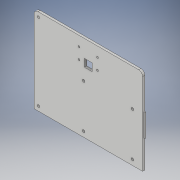
# Autodesk Inventor part: justlid
Saved by Autodesk Inventor 2019 (Build 230136000, 136)
## iProperties
Created: 2019-03-28
Part Number: justlid
Material: Generic
Document SubType Name: Modeling
Designer: eepc07adm
Density: 1 g/cm^3
Appearance: Default
Author: eepc07adm
Autodesk Inventor part; units mm, degrees
ref_plane "YZ Plane" through (0, 0, 0) normal (1, 0, 0) x (0, 1, 0)
ref_plane "XZ Plane" through (0, 0, 0) normal (0, 1, 0) x (-1, 0, 0)
ref_plane "XY Plane" through (0, 0, 0) normal (0, 0, 1) x (1, 0, 0)
sketch "Sketch1" plane through (0, 0, 0) normal (0, 0, 1) x (1, 0, 0)
  line L0 (0, 126.4897) -> (121.92, 126.4897)
  line L1 (121.92, 126.4897) -> (121.92, 29.9697)
  line L2 (121.92, 29.9697) -> (0, 29.9697)
  line L3 (0, 29.9697) -> (0, 126.4897)
  point P0 (0, 0)
  dimension "d0" = 96.52
  dimension "d1" = 121.92
  constraints: 8 end point, 2 parallel, 1 horizontal, 1 perpendicular
  measures "d0" distance between parallel lines of L2 L0
  measures "d1" distance between parallel lines of L3 L1
extrude "Extrusion1" add sketch "Sketch1" along normal blind 2.54
fillet "Fillet1" radius 4.445 1 edges at (0, 126.4897, 1.27)
fillet "Fillet2" radius 4.445 1 edges at (121.92, 126.4897, 1.27)
sketch "Sketch2" plane through (0, 0, 2.54) normal (0, 0, 1) x (1, 0, 0)
  line L0 (56.642, 107.1857) -> (65.278, 107.1857)
  line L1 (65.278, 107.1857) -> (65.278, 98.5497)
  line L2 (65.278, 98.5497) -> (56.642, 98.5497)
  line L3 (56.642, 98.5497) -> (56.642, 107.1857)
  line L4 (121.92, 29.9697) -> (121.92, 122.0447) projected
  line L5 (0, 29.9697) -> (121.92, 29.9697) projected
  point P0 (0, 0)
  dimension "d6" = 8.636
  dimension "d7" = 8.636
  dimension "d8" = 56.642
  dimension "d9" = 68.58
  constraints: 8 end point, 2 parallel, 1 horizontal, 1 perpendicular
  measures "d6" distance between parallel lines of L2 L0
  measures "d7" distance between parallel lines of L1 L3
  measures "d8" distance between parallel lines of L4 L1
  measures "d9" distance between parallel lines of L5 L2
extrude "Extrusion2" cut sketch "Sketch2" against normal blind 2.54
sketch "Sketch3" plane through (0, 0, 2.54) normal (0, 0, 1) x (1, 0, 0)
  line L0 (56.642, 98.5497) -> (56.642, 107.1857) projected
  line L1 (65.278, 107.1857) -> (65.278, 98.5497) projected
  line L2 (56.642, 107.1857) -> (65.278, 107.1857) projected
  point P0 (0, 0)
  point P1 (50.5968, 102.8677)
  point P2 (50.5968, 115.4407)
  point P3 (71.3232, 115.4407)
  point P4 (71.3232, 102.8677)
  dimension "d12" = 6.0452
  dimension "d13" = 6.0452
  dimension "d14" = 12.573
  dimension "d15" = 6.0452
  dimension "d16" = 6.0452
  dimension "d17" = 12.573
  dimension "d27" = 4.318
  dimension "d28" = 4.318
  measures "d12" distance from line of point (50.597, 102.868) L0
  measures "d13" distance from line of point (50.597, 115.441) L0
  measures "d14" distance of point (50.597, 102.868) point (50.597, 115.441)
  measures "d15" distance from line of L1 point (71.323, 115.441)
  measures "d16" distance from line of L1 point (71.323, 102.868)
  measures "d17" distance of point (71.323, 102.868) point (71.323, 115.441)
  measures "d27" distance from line of L2 point (50.597, 102.868)
  measures "d28" distance from line of L2 point (71.323, 102.868)
hole "Hole1" at (50.5968, 115.4407, 2.54) at (71.3232, 115.4407, 2.54) at (71.3232, 102.8677, 2.54) at (50.5968, 102.8677, 2.54) direction (0, 0, -1) diameter 2.0828 end through all
sketch "Sketch4" plane through (0, 0, 2.54) normal (0, 0, 1) x (1, 0, 0)
  line L0 (117.475, 126.4897) -> (4.445, 126.4897) projected
  line L1 (0, 122.0447) -> (0, 29.9697) projected
  line L2 (0, 29.9697) -> (121.92, 29.9697) projected
  point P0 (0, 0)
  point P1 (5.08, 121.4097)
  point P2 (5.08, 35.0497)
  dimension "d29" = 5.08
  dimension "d30" = 5.08
  dimension "d31" = 5.08
  dimension "d32" = 5.08
  measures "d29" distance from line of L0 point (5.08, 121.41)
  measures "d30" distance from line of L1 point (5.08, 121.41)
  measures "d31" distance from line of L2 point (5.08, 35.05)
  measures "d32" distance from line of L1 point (5.08, 35.05)
hole "Hole2" at (5.08, 121.4097, 2.54) at (5.08, 35.0497, 2.54) direction (0, 0, -1) diameter 2.6416 end through all
sketch "Sketch5" plane through (0, 0, 2.54) normal (0, 0, 1) x (1, 0, 0)
  line L0 (52.2478, 88.3389) -> (114.0206, 88.3389)
  line L1 (114.0206, 88.3389) -> (114.0206, 32.4589)
  line L2 (114.0206, 32.4589) -> (52.2478, 32.4589)
  line L3 (52.2478, 32.4589) -> (52.2478, 88.3389)
  line L4 (0, 29.9697) -> (121.92, 29.9697) projected
  line L5 (121.92, 29.9697) -> (121.92, 122.0447) projected
  point P0 (0, 0)
  point P1 (55.7022, 84.8845)
  point P2 (110.5662, 84.8845)
  point P3 (110.5662, 35.9133)
  point P4 (55.7022, 35.9133)
  dimension "d40" = 55.88
  dimension "d41" = 61.7728
  dimension "d42" = 3.4544
  dimension "d43" = 3.4544
  dimension "d44" = 3.4544
  dimension "d45" = 3.4544
  dimension "d46" = 3.4544
  dimension "d47" = 3.4544
  dimension "d48" = 3.4544
  dimension "d49" = 3.4544
  dimension "d50" = 2.4892
  dimension "d51" = 7.8994
  constraints: 8 end point, 2 parallel, 1 horizontal, 1 perpendicular
  measures "d40" distance between parallel lines of L2 L0
  measures "d41" distance between parallel lines of L3 L1
  measures "d42" distance from line of L0 point (55.702, 84.884)
  measures "d43" distance from line of L3 point (55.702, 84.884)
  measures "d44" distance from line of L0 point (110.566, 84.884)
  measures "d45" distance from line of L1 point (110.566, 84.884)
  measures "d46" distance from line of L1 point (110.566, 35.913)
  measures "d47" distance from line of L2 point (110.566, 35.913)
  measures "d48" distance from line of L2 point (55.702, 35.913)
  measures "d49" distance from line of L3 point (55.702, 35.913)
  measures "d50" distance between parallel lines of L4 L2
  measures "d51" distance between parallel lines of L5 L1
hole "Hole3" at (55.7022, 84.8845, 2.54) at (110.5662, 84.8845, 2.54) at (110.5662, 35.9133, 2.54) at (55.7022, 35.9133, 2.54) direction (0, 0, -1) diameter 2.8448 end through all
sketch "Sketch6" plane through (121.92, 29.9697, 2.54) normal (1, 0, 0) x (0, 0, -1)
  line L0 (1.27, 57.15) -> (2.54, 57.15)
  line L1 (2.54, 57.15) -> (2.54, 31.75)
  line L2 (2.54, 31.75) -> (1.27, 31.75)
  line L3 (1.27, 31.75) -> (1.27, 57.15)
  line L4 (2.54, 0) -> (0, 0) projected
  line L5 (0, 0) -> (0, 92.075) projected
  point P0 (2.54, -29.9697)
  dimension "d59" = 25.4
  dimension "d60" = 31.75
  dimension "d61" = 1.27
  dimension "d62" = 1.27
  constraints: 8 end point, 2 parallel, 1 horizontal, 1 perpendicular
  measures "d59" distance between parallel lines of L2 L0
  measures "d60" distance between parallel lines of L4 L2
  measures "d61" distance between parallel lines of L3 L1
  measures "d62" distance between parallel lines of L5 L3
extrude "Extrusion3" add sketch "Sketch6" along normal blind 1.27
body "Solid1"
